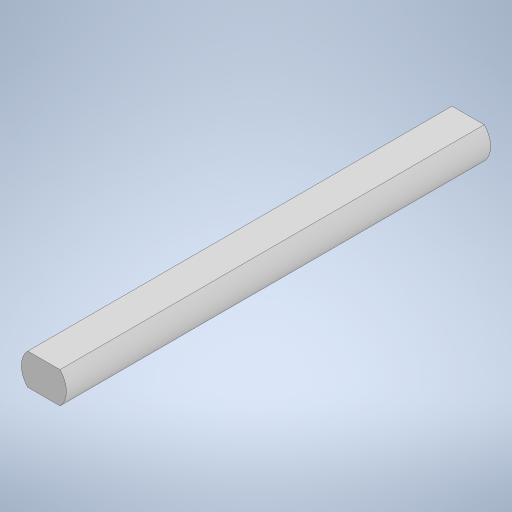
# Autodesk Inventor part: Part1
Saved by Autodesk Inventor 2023.2 (Build 272271000, 271)
## iProperties
Created: 2022-11-25
Part Number: Part1
Material: Generic
Document SubType Name: Modeling
Designer: omrfrkmll
Density: 1 g/cm^3
Appearance: Default
Author: omrfrkmll
Autodesk Inventor part; units mm, degrees
ref_plane "YZ Plane" through (0, 0, 0) normal (1, 0, 0) x (0, 1, 0)
ref_plane "XZ Plane" through (0, 0, 0) normal (0, 1, 0) x (-1, 0, 0)
ref_plane "XY Plane" through (0, 0, 0) normal (0, 0, 1) x (1, 0, 0)
sketch "Sketch1" plane through (0, 0, 0) normal (0, 0, 1) x (1, 0, 0)
  line L0 (-1.8974, 1.85) -> (1.8974, 1.85)
  line L1 (-3.5377, 0) -> (4.2657, 0)
  line L2 (-1.8974, -1.85) -> (1.8974, -1.85)
  arc A0 (-1.8974, 1.85) -> (-1.8974, -1.85) centre (0, 0) ccw
  arc A1 (1.8974, -1.85) -> (1.8974, 1.85) centre (0, 0) ccw
  dimension "d3" = 3.7
  dimension "d6" = 2.65
  dimension "d7" = 2.65
  constraints: 6 end point, 4 horizontal, 4 point on circle, 2 centre point, 1 coincident, 1 other
  measures "d3" distance between parallel lines of L2 L0
  measures "d6" radius of A1
  measures "d7" radius of A0
extrude "Extrusion1" add sketch "Sketch1" along normal blind 50
body "Solid1"
